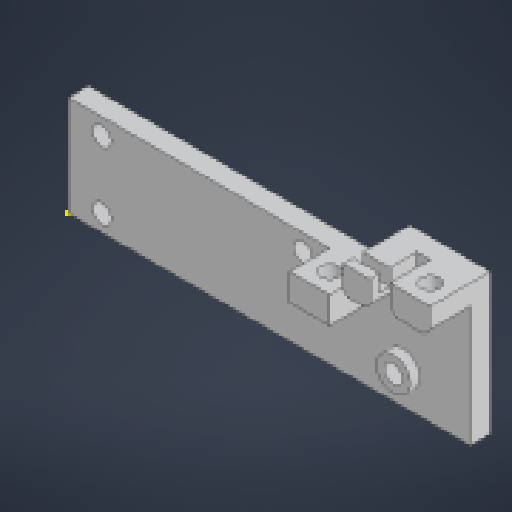
# Autodesk Inventor part: probe mount 1 side
Saved by Autodesk Inventor 2026 (Build 300175050, 175E)
## iProperties
Created: 2025-07-01
Part Number: probe mount 1 side
Material: Generic
Document SubType Name: Modeling
Designer: Tobymegacat
Density: 1 g/cm^3
Appearance: Default
Author: Tobymegacat
Autodesk Inventor part; units mm, degrees
ref_plane "YZ Plane" through (0, 0, 0) normal (1, 0, 0) x (0, 1, 0)
ref_plane "XZ Plane" through (0, 0, 0) normal (0, 1, 0) x (-1, 0, 0)
ref_plane "XY Plane" through (0, 0, 0) normal (0, 0, 1) x (1, 0, 0)
sketch "Sketch1" plane through (0, 0, 0) normal (0, 0, 1) x (1, 0, 0)
  line L0 (0, 0) -> (60, 0)
  line L1 (60, 0) -> (60, 15)
  line L2 (60, 15) -> (0, 15)
  line L3 (0, 15) -> (0, 0)
  dimension "d0" = 60
  dimension "d1" = 15
  constraints: 8 end point, 2 parallel, 1 horizontal, 1 perpendicular
  measures "d0" distance of L2.end L1.end
  measures "d1" distance of L1.end L0.end
extrude "Extrusion1" add sketch "Sketch1" along normal blind 3
sketch "Sketch2" plane through (0, 0, 3) normal (0, 0, 1) x (1, 0, 0)
  line L0 (0, 15) -> (0, 0) projected
  line L1 (0, 0) -> (60, 0) projected
  point P0 (50, 5)
  dimension "d4" = 50
  dimension "d5" = 5
  measures "d4" distance from line of L0 point (50, 5)
  measures "d5" distance from line of L1 point (50, 5)
hole "Hole1" at (50, 5, 3) direction (0, 0, -1) diameter 2.8 depth 10
sketch "Sketch3" plane through (0, 0, 3) normal (0, 0, 1) x (1, 0, 0)
  point P0 (0, 0)
sketch "Sketch4" plane through (0, 0, 3) normal (0, 0, 1) x (1, 0, 0)
  circle A0 centre (50, 5) radius 2.5
  circle A1 centre (50, 5) radius 1.4 projected
  circle A2 centre (50, 5) radius 1.4
  point P0 (0, 0)
  dimension "d13" = 5
  constraints: 2 centre point, 2 concentric, 1 coincident
  measures "d13" diameter of A0
extrude "Extrusion2" add sketch "Sketch4" along normal blind 1.5
sketch "Sketch5" plane through (0, 15, 0) normal (0, 1, 0) x (1, 0, 0)
  line L0 (0, -3) -> (60, -3) projected
  line L1 (60, 0) -> (45, 0)
  line L2 (45, 0) -> (45, -3)
  line L3 (45, -3) -> (60, -3)
  line L4 (60, -3) -> (60, 0)
  point P0 (0, 0)
  dimension "d16" = 15
  constraints: 8 end point, 2 parallel, 1 horizontal, 1 perpendicular, 1 point on line
  measures "d16" distance of L1.start L1.end
extrude "Extrusion3" add sketch "Sketch5" along normal blind 6
sketch "Sketch6" plane through (0, 0, 3) normal (0, 0, 1) x (1, 0, 0)
  line L0 (60, 21) -> (45, 21) projected
  line L1 (48, 21) -> (52, 21)
  line L2 (52, 21) -> (52, 17)
  line L3 (52, 17) -> (48, 17)
  line L4 (48, 17) -> (48, 21)
  line L5 (60, 0) -> (60, 21) projected
  point P0 (0, 0)
  dimension "d19" = 4
  dimension "d20" = 4
  dimension "d21" = 8
  constraints: 8 end point, 2 parallel, 1 horizontal, 1 perpendicular, 1 point on line
  measures "d19" distance of L2.end L3.end
  measures "d20" distance of L1.end L2.end
  measures "d21" distance between parallel lines of L5 L2
extrude "Extrusion4" add sketch "Sketch6" along normal blind 7
sketch "Sketch7" plane through (0, 21, 0) normal (0, 1, 0) x (1, 0, 0)
  line L0 (48, -3) -> (48, -10) projected
  line L1 (52, -3) -> (52, -10) projected
  line L2 (48, -7) -> (52, -7)
  line L3 (52, -7) -> (52, -8.5)
  line L4 (52, -8.5) -> (48, -8.5)
  line L5 (48, -8.5) -> (48, -7)
  line L6 (52, -10) -> (48, -10) projected
  point P0 (0, 0)
  point P1 (50, -8.5)
  dimension "d24" = 1.5
  dimension "d25" = 1.5
  constraints: 8 end point, 2 parallel, 2 point on line, 1 horizontal, 1 midpoint, 1 perpendicular
  measures "d24" distance of L2.end L3.end
  measures "d25" distance from line of L6 point (50, -8.5)
extrude "Extrusion5" cut sketch "Sketch7" against normal blind 2.5 contours L2 L1 L4 L0
sketch "Sketch8" plane through (0, 0, 3) normal (0, 0, 1) x (1, 0, 0)
  line L0 (60, 21) -> (45, 21) projected
  line L1 (60, 21) -> (54, 21)
  line L2 (54, 21) -> (54, 17)
  line L3 (54, 17) -> (60, 17)
  line L4 (60, 17) -> (60, 21)
  point P0 (0, 0)
  dimension "d28" = 6
  dimension "d29" = 4
  constraints: 8 end point, 2 parallel, 1 horizontal, 1 perpendicular
  measures "d28" distance of L3.end L2.end
  measures "d29" distance of L2.end L1.end
extrude "Extrusion6" add sketch "Sketch8" along normal blind 6
sketch "Sketch9" plane through (0, 21, 0) normal (0, 1, 0) x (1, 0, 0)
  line L0 (60, 0) -> (60, -9) projected
  line L1 (60, -9) -> (54, -9) projected
  point P0 (0, 0)
  point P1 (57, -6)
  dimension "d32" = 3
  dimension "d33" = 3
  measures "d32" distance from line of L0 point (57, -6)
  measures "d33" distance from line of L1 point (57, -6)
hole "Hole2" at (57, 21, 6) direction (0, -1, 0) diameter 2.8 depth 5
chamfer "Chamfer1" distance 0.75 angle 45 2 edges at (52, 17, 6.5) (48, 17, 6.5)
chamfer "Chamfer2" distance 1 angle 45 2 edges at (60, 17, 6) (54, 17, 6)
chamfer "Chamfer3" distance 3 distance2 6 1 edges at (45, 21, 1.5) measured on face at (53, 21, 1)
sketch "Sketch10" plane through (0, 0, 3) normal (0, 0, 1) x (1, 0, 0)
  line L0 (45, 15) -> (0, 15) projected
  line L1 (45, 15) -> (39, 15)
  line L2 (39, 15) -> (39, 11)
  line L3 (39, 11) -> (45, 11)
  line L4 (45, 11) -> (45, 15)
  point P0 (0, 0)
  dimension "d50" = 6
  dimension "d51" = 4
  constraints: 8 end point, 2 parallel, 1 horizontal, 1 perpendicular
  measures "d50" distance of L3.end L2.end
  measures "d51" distance of L2.end L1.end
extrude "Extrusion7" add sketch "Sketch10" along normal blind 6
sketch "Sketch11" plane through (0, 15, 3) normal (0, 1, 0) x (1, 0, 0)
  line L0 (45, -6) -> (39, -6) projected
  line L1 (39, 0) -> (39, -6) projected
  point P0 (0, 3)
  point P1 (42, -3)
  dimension "d54" = 3
  dimension "d55" = 3
  measures "d54" distance from line of L0 point (42, -3)
  measures "d55" distance from line of L1 point (42, -3)
hole "Hole3" at (42, 15, 6) direction (0, -1, 0) diameter 2.8 depth 5
sketch "Sketch12" plane through (0, 0, 3) normal (0, 0, 1) x (1, 0, 0)
  line L0 (35, 12.5) -> (5, 12.5)
  line L1 (5, 12.5) -> (5, 2.5)
  line L2 (12.2868, 12.5) -> (12.2868, 15)
  line L3 (45, 15) -> (0, 15) projected
  line L4 (11.9839, 2.5) -> (11.9839, 0)
  line L5 (0, 0) -> (60, 0) projected
  line L6 (0, 15) -> (0, 0) projected
  dimension "d64" = 10
  dimension "d65" = 5
  constraints: 8 end point, 3 point on line, 3 vertical, 2 horizontal, 1 horizontal alignment, 1 parallel, 1 perpendicular, 4 other
  measures "d64" distance of L1.end L0.end
  measures "d65" distance between parallel lines of L6 L1
hole "Hole4" at (35, 12.5, 3) at (5, 12.5, 3) at (5, 2.5, 3) direction (0, 0, -1) diameter 2.8 depth 3
body "Solid1"
